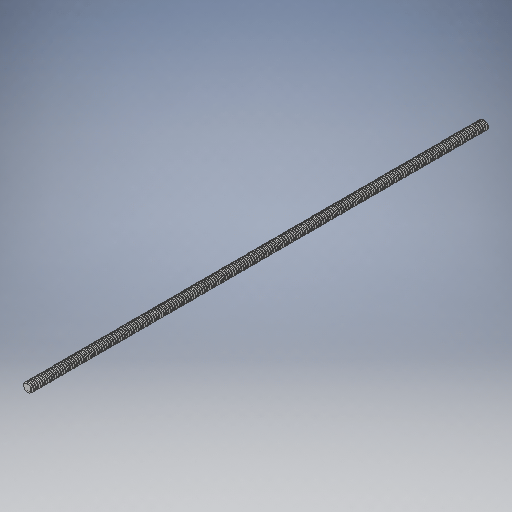
# Autodesk Inventor part: Lead screw 2pitch_8lead_400mm
Saved by Autodesk Inventor 2025.2 (Build 292293000, 293)
## iProperties
Created: 2025-04-06
Part Number: Lead screw 2pitch_8lead_400mm
Material: Generic
Document SubType Name: Modeling
Designer: Tiago
Density: 1 g/cm^3
Appearance: Default
Author: Tiago
Autodesk Inventor part; units mm, degrees
ref_plane "YZ Plane" through (0, 0, 0) normal (1, 0, 0) x (0, 1, 0)
ref_plane "XZ Plane" through (0, 0, 0) normal (0, 1, 0) x (-1, 0, 0)
ref_plane "XY Plane" through (0, 0, 0) normal (0, 0, 1) x (1, 0, 0)
sketch "Sketch1" plane through (0, 0, 0) normal (0, 0, 1) x (1, 0, 0)
  circle A0 centre (0, 0) radius 4
  dimension "Base" = 8
  constraints: 1 centre point, 1 coincident
  measures "Base" diameter of A0
extrude "Extrusion1" add sketch "Sketch1" along normal blind 400
chamfer "Chamfer1" distance 0.3 angle 45 1 edges at (-4, 0, 400)
sketch "Sketch2" plane through (0, 0, 0) normal (0, 1, 0) x (-1, 0, 0)
  line L0 (-4, 399.7) -> (-3.7, 400) projected
  line L1 (-3.7, 400) -> (3.7, 400) projected
  line L2 (3.7, 400) -> (4, 399.7) projected
  line L3 (4, 399.7) -> (4, 0) projected
  line L4 (4, 0) -> (-4, 0) projected
  line L5 (-4, 0) -> (-4, 399.7) projected
  line L6 (4, 400.6339) -> (2.75, 400.6339) construction
  line L7 (2.75, 400.9329) -> (2.75, 400.3349)
  line L8 (4, 401.2679) -> (4, 400)
  line L9 (2.75, 400.3349) -> (4, 400)
  line L10 (2.75, 400.9329) -> (4, 401.2679)
  line L11 (0, 402.735) -> (0, 397.4381) construction
  line L12 (-4, 400.6339) -> (-2.75, 400.6339) construction
  line L13 (-2.75, 400.9329) -> (-2.75, 400.3349)
  line L14 (-4, 401.2679) -> (-4, 400)
  line L15 (-2.75, 400.3349) -> (-4, 400)
  line L16 (-2.75, 400.9329) -> (-4, 401.2679)
  point P0 (0, 0)
  dimension "di" = 1.25
  dimension "d8" = 0.598
  dimension "d12" = 30
  constraints: 22 end point, 6 symmetric about line, 1 collinear, 1 midpoint, 1 parallel, 1 vertical
  measures "di" distance of L6.start L6.end
  measures "d8" distance of L7.start L7.end
  measures "d12" angle of L10 L9
coil "Coil1" sketch "Sketch2" operation cut axis through (0, 0, -10) along (0, 0, -1) pitch 2 turns 202.5 hand right contours L10 L8 L9 L7
sketch "Sketch3" plane through (0, 0, 0) normal (1, 0, 0) x (0, 1, 0)
  line L0 (2.75, 0.4329) -> (2.75, 0) projected
  line L1 (2.75, 0) -> (-4, 0) projected
  line L2 (-2.75, 398.8349) -> (-2.75, 399.4329) projected
  line L3 (-3.7, 400) -> (2.75, 400) projected
  line L4 (2.75, 400) -> (2.75, 399.8349) projected
  line L5 (-2.75, 0.8349) -> (-2.75, 1.4329) projected
  line L6 (-2.75, 2.8349) -> (-2.75, 3.4329) projected
  line L7 (-2.75, 4.8349) -> (-2.75, 5.4329) projected
  line L8 (-2.75, 6.8349) -> (-2.75, 7.4329) projected
  line L9 (-2.75, 8.8349) -> (-2.75, 9.4329) projected
  line L10 (-2.75, 10.8349) -> (-2.75, 11.4329) projected
  line L11 (-2.75, 12.8349) -> (-2.75, 13.4329) projected
  line L12 (-2.75, 14.8349) -> (-2.75, 15.4329) projected
  line L13 (-2.75, 16.8349) -> (-2.75, 17.4329) projected
  line L14 (-2.75, 18.8349) -> (-2.75, 19.4329) projected
  line L15 (-2.75, 20.8349) -> (-2.75, 21.4329) projected
  line L16 (-2.75, 22.8349) -> (-2.75, 23.4329) projected
  line L17 (-2.75, 24.8349) -> (-2.75, 25.4329) projected
  line L18 (-2.75, 26.8349) -> (-2.75, 27.4329) projected
  line L19 (-2.75, 28.8349) -> (-2.75, 29.4329) projected
  line L20 (-2.75, 30.8349) -> (-2.75, 31.4329) projected
  line L21 (-2.75, 32.8349) -> (-2.75, 33.4329) projected
  line L22 (-2.75, 34.8349) -> (-2.75, 35.4329) projected
  line L23 (-2.75, 36.8349) -> (-2.75, 37.4329) projected
  line L24 (-2.75, 38.8349) -> (-2.75, 39.4329) projected
  line L25 (-2.75, 40.8349) -> (-2.75, 41.4329) projected
  line L26 (-2.75, 42.8349) -> (-2.75, 43.4329) projected
  line L27 (-2.75, 44.8349) -> (-2.75, 45.4329) projected
  line L28 (-2.75, 46.8349) -> (-2.75, 47.4329) projected
  line L29 (-2.75, 48.8349) -> (-2.75, 49.4329) projected
  line L30 (-2.75, 50.8349) -> (-2.75, 51.4329) projected
  line L31 (-2.75, 52.8349) -> (-2.75, 53.4329) projected
  line L32 (-2.75, 54.8349) -> (-2.75, 55.4329) projected
  line L33 (-2.75, 56.8349) -> (-2.75, 57.4329) projected
  line L34 (-2.75, 58.8349) -> (-2.75, 59.4329) projected
  line L35 (-2.75, 60.8349) -> (-2.75, 61.4329) projected
  line L36 (-2.75, 62.8349) -> (-2.75, 63.4329) projected
  line L37 (-2.75, 64.8349) -> (-2.75, 65.4329) projected
  line L38 (-2.75, 66.8349) -> (-2.75, 67.4329) projected
  line L39 (-2.75, 68.8349) -> (-2.75, 69.4329) projected
  line L40 (-2.75, 70.8349) -> (-2.75, 71.4329) projected
  line L41 (-2.75, 72.8349) -> (-2.75, 73.4329) projected
  line L42 (-2.75, 74.8349) -> (-2.75, 75.4329) projected
  line L43 (-2.75, 76.8349) -> (-2.75, 77.4329) projected
  line L44 (-2.75, 78.8349) -> (-2.75, 79.4329) projected
  line L45 (-2.75, 80.8349) -> (-2.75, 81.4329) projected
  line L46 (-2.75, 82.8349) -> (-2.75, 83.4329) projected
  line L47 (-2.75, 84.8349) -> (-2.75, 85.4329) projected
  line L48 (-2.75, 86.8349) -> (-2.75, 87.4329) projected
  line L49 (-2.75, 88.8349) -> (-2.75, 89.4329) projected
  line L50 (-2.75, 90.8349) -> (-2.75, 91.4329) projected
  line L51 (-2.75, 92.8349) -> (-2.75, 93.4329) projected
  line L52 (-2.75, 94.8349) -> (-2.75, 95.4329) projected
  line L53 (-2.75, 96.8349) -> (-2.75, 97.4329) projected
  line L54 (-2.75, 98.8349) -> (-2.75, 99.4329) projected
  line L55 (-2.75, 100.8349) -> (-2.75, 101.4329) projected
  line L56 (-2.75, 102.8349) -> (-2.75, 103.4329) projected
  line L57 (-2.75, 104.8349) -> (-2.75, 105.4329) projected
  line L58 (-2.75, 106.8349) -> (-2.75, 107.4329) projected
  line L59 (-2.75, 108.8349) -> (-2.75, 109.4329) projected
  line L60 (-2.75, 110.8349) -> (-2.75, 111.4329) projected
  line L61 (-2.75, 112.8349) -> (-2.75, 113.4329) projected
  line L62 (-2.75, 114.8349) -> (-2.75, 115.4329) projected
  line L63 (-2.75, 116.8349) -> (-2.75, 117.4329) projected
  line L64 (-2.75, 118.8349) -> (-2.75, 119.4329) projected
  line L65 (-2.75, 120.8349) -> (-2.75, 121.4329) projected
  line L66 (-2.75, 122.8349) -> (-2.75, 123.4329) projected
  line L67 (-2.75, 124.8349) -> (-2.75, 125.4329) projected
  line L68 (-2.75, 126.8349) -> (-2.75, 127.4329) projected
  line L69 (-2.75, 128.8349) -> (-2.75, 129.4329) projected
  line L70 (-2.75, 130.8349) -> (-2.75, 131.4329) projected
  line L71 (-2.75, 132.8349) -> (-2.75, 133.4329) projected
  line L72 (-2.75, 134.8349) -> (-2.75, 135.4329) projected
  line L73 (-2.75, 136.8349) -> (-2.75, 137.4329) projected
  line L74 (-2.75, 138.8349) -> (-2.75, 139.4329) projected
  line L75 (-2.75, 140.8349) -> (-2.75, 141.4329) projected
  line L76 (-2.75, 142.8349) -> (-2.75, 143.4329) projected
  line L77 (-2.75, 144.8349) -> (-2.75, 145.4329) projected
  line L78 (-2.75, 146.8349) -> (-2.75, 147.4329) projected
  line L79 (-2.75, 148.8349) -> (-2.75, 149.4329) projected
  line L80 (-2.75, 150.8349) -> (-2.75, 151.4329) projected
  line L81 (-2.75, 152.8349) -> (-2.75, 153.4329) projected
  line L82 (-2.75, 154.8349) -> (-2.75, 155.4329) projected
  line L83 (-2.75, 156.8349) -> (-2.75, 157.4329) projected
  line L84 (-2.75, 158.8349) -> (-2.75, 159.4329) projected
  line L85 (-2.75, 160.8349) -> (-2.75, 161.4329) projected
  line L86 (-2.75, 162.8349) -> (-2.75, 163.4329) projected
  line L87 (-2.75, 164.8349) -> (-2.75, 165.4329) projected
  line L88 (-2.75, 166.8349) -> (-2.75, 167.4329) projected
  line L89 (-2.75, 168.8349) -> (-2.75, 169.4329) projected
  line L90 (-2.75, 170.8349) -> (-2.75, 171.4329) projected
  line L91 (-2.75, 172.8349) -> (-2.75, 173.4329) projected
  line L92 (-2.75, 174.8349) -> (-2.75, 175.4329) projected
  line L93 (-2.75, 176.8349) -> (-2.75, 177.4329) projected
  line L94 (-2.75, 178.8349) -> (-2.75, 179.4329) projected
  line L95 (-2.75, 180.8349) -> (-2.75, 181.4329) projected
  line L96 (-2.75, 182.8349) -> (-2.75, 183.4329) projected
  line L97 (-2.75, 184.8349) -> (-2.75, 185.4329) projected
  line L98 (-2.75, 186.8349) -> (-2.75, 187.4329) projected
  line L99 (-2.75, 188.8349) -> (-2.75, 189.4329) projected
  line L100 (-2.75, 190.8349) -> (-2.75, 191.4329) projected
  line L101 (-2.75, 192.8349) -> (-2.75, 193.4329) projected
  line L102 (-2.75, 194.8349) -> (-2.75, 195.4329) projected
  line L103 (-2.75, 196.8349) -> (-2.75, 197.4329) projected
  line L104 (-2.75, 198.8349) -> (-2.75, 199.4329) projected
  line L105 (-2.75, 200.8349) -> (-2.75, 201.4329) projected
  line L106 (-2.75, 202.8349) -> (-2.75, 203.4329) projected
  line L107 (-2.75, 204.8349) -> (-2.75, 205.4329) projected
  line L108 (-2.75, 206.8349) -> (-2.75, 207.4329) projected
  line L109 (-2.75, 208.8349) -> (-2.75, 209.4329) projected
  line L110 (-2.75, 210.8349) -> (-2.75, 211.4329) projected
  line L111 (-2.75, 212.8349) -> (-2.75, 213.4329) projected
  line L112 (-2.75, 214.8349) -> (-2.75, 215.4329) projected
  line L113 (-2.75, 216.8349) -> (-2.75, 217.4329) projected
  line L114 (-2.75, 218.8349) -> (-2.75, 219.4329) projected
  line L115 (-2.75, 220.8349) -> (-2.75, 221.4329) projected
  line L116 (-2.75, 222.8349) -> (-2.75, 223.4329) projected
  line L117 (-2.75, 224.8349) -> (-2.75, 225.4329) projected
  line L118 (-2.75, 226.8349) -> (-2.75, 227.4329) projected
  line L119 (-2.75, 228.8349) -> (-2.75, 229.4329) projected
  line L120 (-2.75, 230.8349) -> (-2.75, 231.4329) projected
  line L121 (-2.75, 232.8349) -> (-2.75, 233.4329) projected
  line L122 (-2.75, 234.8349) -> (-2.75, 235.4329) projected
  line L123 (-2.75, 236.8349) -> (-2.75, 237.4329) projected
  line L124 (-2.75, 238.8349) -> (-2.75, 239.4329) projected
  line L125 (-2.75, 240.8349) -> (-2.75, 241.4329) projected
  line L126 (-2.75, 242.8349) -> (-2.75, 243.4329) projected
  line L127 (-2.75, 244.8349) -> (-2.75, 245.4329) projected
  line L128 (-2.75, 246.8349) -> (-2.75, 247.4329) projected
  line L129 (-2.75, 248.8349) -> (-2.75, 249.4329) projected
  line L130 (-2.75, 250.8349) -> (-2.75, 251.4329) projected
  line L131 (-2.75, 252.8349) -> (-2.75, 253.4329) projected
  line L132 (-2.75, 254.8349) -> (-2.75, 255.4329) projected
  line L133 (-2.75, 256.8349) -> (-2.75, 257.4329) projected
  line L134 (-2.75, 258.8349) -> (-2.75, 259.4329) projected
  line L135 (-2.75, 260.8349) -> (-2.75, 261.4329) projected
  line L136 (-2.75, 262.8349) -> (-2.75, 263.4329) projected
  line L137 (-2.75, 264.8349) -> (-2.75, 265.4329) projected
  line L138 (-2.75, 266.8349) -> (-2.75, 267.4329) projected
  line L139 (-2.75, 268.8349) -> (-2.75, 269.4329) projected
  line L140 (-2.75, 270.8349) -> (-2.75, 271.4329) projected
  line L141 (-2.75, 272.8349) -> (-2.75, 273.4329) projected
  line L142 (-2.75, 274.8349) -> (-2.75, 275.4329) projected
  line L143 (-2.75, 276.8349) -> (-2.75, 277.4329) projected
  line L144 (-2.75, 278.8349) -> (-2.75, 279.4329) projected
  line L145 (-2.75, 280.8349) -> (-2.75, 281.4329) projected
  line L146 (-2.75, 282.8349) -> (-2.75, 283.4329) projected
  line L147 (-2.75, 284.8349) -> (-2.75, 285.4329) projected
  line L148 (-2.75, 286.8349) -> (-2.75, 287.4329) projected
  line L149 (-2.75, 288.8349) -> (-2.75, 289.4329) projected
  line L150 (-2.75, 290.8349) -> (-2.75, 291.4329) projected
  line L151 (-2.75, 292.8349) -> (-2.75, 293.4329) projected
  line L152 (-2.75, 294.8349) -> (-2.75, 295.4329) projected
  line L153 (-2.75, 296.8349) -> (-2.75, 297.4329) projected
  line L154 (-2.75, 298.8349) -> (-2.75, 299.4329) projected
  line L155 (-2.75, 300.8349) -> (-2.75, 301.4329) projected
  line L156 (-2.75, 302.8349) -> (-2.75, 303.4329) projected
  line L157 (-2.75, 304.8349) -> (-2.75, 305.4329) projected
  line L158 (-2.75, 306.8349) -> (-2.75, 307.4329) projected
  line L159 (-2.75, 308.8349) -> (-2.75, 309.4329) projected
  line L160 (-2.75, 310.8349) -> (-2.75, 311.4329) projected
  line L161 (-2.75, 312.8349) -> (-2.75, 313.4329) projected
  line L162 (-2.75, 314.8349) -> (-2.75, 315.4329) projected
  line L163 (-2.75, 316.8349) -> (-2.75, 317.4329) projected
  line L164 (-2.75, 318.8349) -> (-2.75, 319.4329) projected
  line L165 (-2.75, 320.8349) -> (-2.75, 321.4329) projected
  line L166 (-2.75, 322.8349) -> (-2.75, 323.4329) projected
  line L167 (-2.75, 324.8349) -> (-2.75, 325.4329) projected
  line L168 (-2.75, 326.8349) -> (-2.75, 327.4329) projected
  line L169 (-2.75, 328.8349) -> (-2.75, 329.4329) projected
  line L170 (-2.75, 330.8349) -> (-2.75, 331.4329) projected
  line L171 (-2.75, 332.8349) -> (-2.75, 333.4329) projected
  line L172 (-2.75, 334.8349) -> (-2.75, 335.4329) projected
  line L173 (-2.75, 336.8349) -> (-2.75, 337.4329) projected
  line L174 (-2.75, 338.8349) -> (-2.75, 339.4329) projected
  line L175 (-2.75, 340.8349) -> (-2.75, 341.4329) projected
  line L176 (-2.75, 342.8349) -> (-2.75, 343.4329) projected
  line L177 (-2.75, 344.8349) -> (-2.75, 345.4329) projected
  line L178 (-2.75, 346.8349) -> (-2.75, 347.4329) projected
  line L179 (-2.75, 348.8349) -> (-2.75, 349.4329) projected
  line L180 (-2.75, 350.8349) -> (-2.75, 351.4329) projected
  line L181 (-2.75, 352.8349) -> (-2.75, 353.4329) projected
  line L182 (-2.75, 354.8349) -> (-2.75, 355.4329) projected
  line L183 (-2.75, 356.8349) -> (-2.75, 357.4329) projected
  line L184 (-2.75, 358.8349) -> (-2.75, 359.4329) projected
  line L185 (-2.75, 360.8349) -> (-2.75, 361.4329) projected
  line L186 (-2.75, 362.8349) -> (-2.75, 363.4329) projected
  line L187 (-2.75, 364.8349) -> (-2.75, 365.4329) projected
  line L188 (-2.75, 366.8349) -> (-2.75, 367.4329) projected
  line L189 (-2.75, 368.8349) -> (-2.75, 369.4329) projected
  line L190 (-2.75, 370.8349) -> (-2.75, 371.4329) projected
  line L191 (-2.75, 372.8349) -> (-2.75, 373.4329) projected
  line L192 (-2.75, 374.8349) -> (-2.75, 375.4329) projected
  line L193 (-2.75, 376.8349) -> (-2.75, 377.4329) projected
  line L194 (-2.75, 378.8349) -> (-2.75, 379.4329) projected
  line L195 (-2.75, 380.8349) -> (-2.75, 381.4329) projected
  line L196 (-2.75, 382.8349) -> (-2.75, 383.4329) projected
  line L197 (-2.75, 384.8349) -> (-2.75, 385.4329) projected
  line L198 (-2.75, 386.8349) -> (-2.75, 387.4329) projected
  line L199 (-2.75, 388.8349) -> (-2.75, 389.4329) projected
  line L200 (-2.75, 390.8349) -> (-2.75, 391.4329) projected
  line L201 (-2.75, 392.8349) -> (-2.75, 393.4329) projected
  line L202 (-2.75, 394.8349) -> (-2.75, 395.4329) projected
  line L203 (-2.75, 396.8349) -> (-2.75, 397.4329) projected
  line L204 (2.7534, 400.6412) -> (4.0034, 400.6412) construction
  line L205 (4.0034, 400.9402) -> (4.0034, 400.3422)
  line L206 (2.7534, 401.2752) -> (2.7534, 400.0073)
  line L207 (4.0034, 400.3422) -> (2.7534, 400.0073)
  line L208 (4.0034, 400.9402) -> (2.7534, 401.2752)
  line L209 (0, 399.0551) -> (0, 402.6988)
  line L210 (-3.9465, 399.7535) -> (-3.7, 400) projected
  line L211 (4, 399.5) -> (4, 398.7679) projected
  line L212 (2.75, 398.4329) -> (2.75, 397.8349) projected
  line L213 (4, 397.5) -> (4, 396.7679) projected
  line L214 (2.75, 396.4329) -> (2.75, 395.8349) projected
  line L215 (4, 395.5) -> (4, 394.7679) projected
  line L216 (2.75, 394.4329) -> (2.75, 393.8349) projected
  line L217 (4, 393.5) -> (4, 392.7679) projected
  line L218 (2.75, 392.4329) -> (2.75, 391.8349) projected
  line L219 (4, 391.5) -> (4, 390.7679) projected
  line L220 (2.75, 390.4329) -> (2.75, 389.8349) projected
  line L221 (4, 389.5) -> (4, 388.7679) projected
  line L222 (2.75, 388.4329) -> (2.75, 387.8349) projected
  line L223 (4, 387.5) -> (4, 386.7679) projected
  line L224 (2.75, 386.4329) -> (2.75, 385.8349) projected
  line L225 (4, 385.5) -> (4, 384.7679) projected
  line L226 (2.75, 384.4329) -> (2.75, 383.8349) projected
  line L227 (4, 383.5) -> (4, 382.7679) projected
  line L228 (2.75, 382.4329) -> (2.75, 381.8349) projected
  line L229 (4, 381.5) -> (4, 380.7679) projected
  line L230 (2.75, 380.4329) -> (2.75, 379.8349) projected
  line L231 (4, 379.5) -> (4, 378.7679) projected
  line L232 (2.75, 378.4329) -> (2.75, 377.8349) projected
  line L233 (4, 377.5) -> (4, 376.7679) projected
  line L234 (2.75, 376.4329) -> (2.75, 375.8349) projected
  line L235 (4, 375.5) -> (4, 374.7679) projected
  line L236 (2.75, 374.4329) -> (2.75, 373.8349) projected
  line L237 (4, 373.5) -> (4, 372.7679) projected
  line L238 (2.75, 372.4329) -> (2.75, 371.8349) projected
  line L239 (4, 371.5) -> (4, 370.7679) projected
  line L240 (2.75, 370.4329) -> (2.75, 369.8349) projected
  line L241 (4, 369.5) -> (4, 368.7679) projected
  line L242 (2.75, 368.4329) -> (2.75, 367.8349) projected
  line L243 (4, 367.5) -> (4, 366.7679) projected
  line L244 (2.75, 366.4329) -> (2.75, 365.8349) projected
  line L245 (4, 365.5) -> (4, 364.7679) projected
  line L246 (2.75, 364.4329) -> (2.75, 363.8349) projected
  line L247 (4, 363.5) -> (4, 362.7679) projected
  line L248 (2.75, 362.4329) -> (2.75, 361.8349) projected
  line L249 (4, 361.5) -> (4, 360.7679) projected
  line L250 (2.75, 360.4329) -> (2.75, 359.8349) projected
  line L251 (4, 359.5) -> (4, 358.7679) projected
  line L252 (2.75, 358.4329) -> (2.75, 357.8349) projected
  line L253 (4, 357.5) -> (4, 356.7679) projected
  line L254 (2.75, 356.4329) -> (2.75, 355.8349) projected
  line L255 (4, 355.5) -> (4, 354.7679) projected
  line L256 (2.75, 354.4329) -> (2.75, 353.8349) projected
  line L257 (4, 353.5) -> (4, 352.7679) projected
  line L258 (2.75, 352.4329) -> (2.75, 351.8349) projected
  line L259 (4, 351.5) -> (4, 350.7679) projected
  line L260 (2.75, 350.4329) -> (2.75, 349.8349) projected
  line L261 (4, 349.5) -> (4, 348.7679) projected
  line L262 (2.75, 348.4329) -> (2.75, 347.8349) projected
  line L263 (4, 347.5) -> (4, 346.7679) projected
  line L264 (2.75, 346.4329) -> (2.75, 345.8349) projected
  line L265 (4, 345.5) -> (4, 344.7679) projected
  line L266 (2.75, 344.4329) -> (2.75, 343.8349) projected
  line L267 (4, 343.5) -> (4, 342.7679) projected
  line L268 (2.75, 342.4329) -> (2.75, 341.8349) projected
  line L269 (4, 341.5) -> (4, 340.7679) projected
  line L270 (2.75, 340.4329) -> (2.75, 339.8349) projected
  line L271 (4, 339.5) -> (4, 338.7679) projected
  line L272 (2.75, 338.4329) -> (2.75, 337.8349) projected
  line L273 (4, 337.5) -> (4, 336.7679) projected
  line L274 (2.75, 336.4329) -> (2.75, 335.8349) projected
  line L275 (4, 335.5) -> (4, 334.7679) projected
  line L276 (2.75, 334.4329) -> (2.75, 333.8349) projected
  line L277 (4, 333.5) -> (4, 332.7679) projected
  line L278 (2.75, 332.4329) -> (2.75, 331.8349) projected
  line L279 (4, 331.5) -> (4, 330.7679) projected
  line L280 (2.75, 330.4329) -> (2.75, 329.8349) projected
  line L281 (4, 329.5) -> (4, 328.7679) projected
  line L282 (2.75, 328.4329) -> (2.75, 327.8349) projected
  line L283 (4, 327.5) -> (4, 326.7679) projected
  line L284 (2.75, 326.4329) -> (2.75, 325.8349) projected
  line L285 (4, 325.5) -> (4, 324.7679) projected
  line L286 (2.75, 324.4329) -> (2.75, 323.8349) projected
  line L287 (4, 323.5) -> (4, 322.7679) projected
  line L288 (2.75, 322.4329) -> (2.75, 321.8349) projected
  line L289 (4, 321.5) -> (4, 320.7679) projected
  line L290 (2.75, 320.4329) -> (2.75, 319.8349) projected
  line L291 (4, 319.5) -> (4, 318.7679) projected
  line L292 (2.75, 318.4329) -> (2.75, 317.8349) projected
  line L293 (4, 317.5) -> (4, 316.7679) projected
  line L294 (2.75, 316.4329) -> (2.75, 315.8349) projected
  line L295 (4, 315.5) -> (4, 314.7679) projected
  line L296 (2.75, 314.4329) -> (2.75, 313.8349) projected
  line L297 (4, 313.5) -> (4, 312.7679) projected
  line L298 (2.75, 312.4329) -> (2.75, 311.8349) projected
  line L299 (4, 311.5) -> (4, 310.7679) projected
  line L300 (2.75, 310.4329) -> (2.75, 309.8349) projected
  line L301 (4, 309.5) -> (4, 308.7679) projected
  line L302 (2.75, 308.4329) -> (2.75, 307.8349) projected
  line L303 (4, 307.5) -> (4, 306.7679) projected
  line L304 (2.75, 306.4329) -> (2.75, 305.8349) projected
  line L305 (4, 305.5) -> (4, 304.7679) projected
  line L306 (2.75, 304.4329) -> (2.75, 303.8349) projected
  line L307 (4, 303.5) -> (4, 302.7679) projected
  line L308 (2.75, 302.4329) -> (2.75, 301.8349) projected
  line L309 (4, 301.5) -> (4, 300.7679) projected
  line L310 (2.75, 300.4329) -> (2.75, 299.8349) projected
  line L311 (4, 299.5) -> (4, 298.7679) projected
  line L312 (2.75, 298.4329) -> (2.75, 297.8349) projected
  line L313 (4, 297.5) -> (4, 296.7679) projected
  line L314 (2.75, 296.4329) -> (2.75, 295.8349) projected
  line L315 (4, 295.5) -> (4, 294.7679) projected
  line L316 (2.75, 294.4329) -> (2.75, 293.8349) projected
  line L317 (4, 293.5) -> (4, 292.7679) projected
  line L318 (2.75, 292.4329) -> (2.75, 291.8349) projected
  line L319 (4, 291.5) -> (4, 290.7679) projected
  line L320 (2.75, 290.4329) -> (2.75, 289.8349) projected
  line L321 (4, 289.5) -> (4, 288.7679) projected
  line L322 (2.75, 288.4329) -> (2.75, 287.8349) projected
  line L323 (4, 287.5) -> (4, 286.7679) projected
  line L324 (2.75, 286.4329) -> (2.75, 285.8349) projected
  line L325 (4, 285.5) -> (4, 284.7679) projected
  line L326 (2.75, 284.4329) -> (2.75, 283.8349) projected
  line L327 (4, 283.5) -> (4, 282.7679) projected
  line L328 (2.75, 282.4329) -> (2.75, 281.8349) projected
  line L329 (4, 281.5) -> (4, 280.7679) projected
  line L330 (2.75, 280.4329) -> (2.75, 279.8349) projected
  line L331 (4, 279.5) -> (4, 278.7679) projected
  line L332 (2.75, 278.4329) -> (2.75, 277.8349) projected
  line L333 (4, 277.5) -> (4, 276.7679) projected
  line L334 (2.75, 276.4329) -> (2.75, 275.8349) projected
  line L335 (4, 275.5) -> (4, 274.7679) projected
  line L336 (2.75, 274.4329) -> (2.75, 273.8349) projected
  line L337 (4, 273.5) -> (4, 272.7679) projected
  line L338 (2.75, 272.4329) -> (2.75, 271.8349) projected
  line L339 (4, 271.5) -> (4, 270.7679) projected
  line L340 (2.75, 270.4329) -> (2.75, 269.8349) projected
  line L341 (4, 269.5) -> (4, 268.7679) projected
  line L342 (2.75, 268.4329) -> (2.75, 267.8349) projected
  line L343 (4, 267.5) -> (4, 266.7679) projected
  line L344 (2.75, 266.4329) -> (2.75, 265.8349) projected
  line L345 (4, 265.5) -> (4, 264.7679) projected
  line L346 (2.75, 264.4329) -> (2.75, 263.8349) projected
  line L347 (4, 263.5) -> (4, 262.7679) projected
  line L348 (2.75, 262.4329) -> (2.75, 261.8349) projected
  line L349 (4, 261.5) -> (4, 260.7679) projected
  line L350 (2.75, 260.4329) -> (2.75, 259.8349) projected
  line L351 (4, 259.5) -> (4, 258.7679) projected
  line L352 (2.75, 258.4329) -> (2.75, 257.8349) projected
  line L353 (4, 257.5) -> (4, 256.7679) projected
  line L354 (2.75, 256.4329) -> (2.75, 255.8349) projected
  line L355 (4, 255.5) -> (4, 254.7679) projected
  line L356 (2.75, 254.4329) -> (2.75, 253.8349) projected
  line L357 (4, 253.5) -> (4, 252.7679) projected
  line L358 (2.75, 252.4329) -> (2.75, 251.8349) projected
  line L359 (4, 251.5) -> (4, 250.7679) projected
  line L360 (2.75, 250.4329) -> (2.75, 249.8349) projected
  line L361 (4, 249.5) -> (4, 248.7679) projected
  line L362 (2.75, 248.4329) -> (2.75, 247.8349) projected
  line L363 (4, 247.5) -> (4, 246.7679) projected
  line L364 (2.75, 246.4329) -> (2.75, 245.8349) projected
  line L365 (4, 245.5) -> (4, 244.7679) projected
  line L366 (2.75, 244.4329) -> (2.75, 243.8349) projected
  line L367 (4, 243.5) -> (4, 242.7679) projected
  line L368 (2.75, 242.4329) -> (2.75, 241.8349) projected
  line L369 (4, 241.5) -> (4, 240.7679) projected
  line L370 (2.75, 240.4329) -> (2.75, 239.8349) projected
  line L371 (4, 239.5) -> (4, 238.7679) projected
  line L372 (2.75, 238.4329) -> (2.75, 237.8349) projected
  line L373 (4, 237.5) -> (4, 236.7679) projected
  line L374 (2.75, 236.4329) -> (2.75, 235.8349) projected
  line L375 (4, 235.5) -> (4, 234.7679) projected
  line L376 (2.75, 234.4329) -> (2.75, 233.8349) projected
  line L377 (4, 233.5) -> (4, 232.7679) projected
  line L378 (2.75, 232.4329) -> (2.75, 231.8349) projected
  line L379 (4, 231.5) -> (4, 230.7679) projected
  line L380 (2.75, 230.4329) -> (2.75, 229.8349) projected
  line L381 (4, 229.5) -> (4, 228.7679) projected
  line L382 (2.75, 228.4329) -> (2.75, 227.8349) projected
  line L383 (4, 227.5) -> (4, 226.7679) projected
  line L384 (2.75, 226.4329) -> (2.75, 225.8349) projected
  line L385 (4, 225.5) -> (4, 224.7679) projected
  line L386 (2.75, 224.4329) -> (2.75, 223.8349) projected
  line L387 (4, 223.5) -> (4, 222.7679) projected
  line L388 (2.75, 222.4329) -> (2.75, 221.8349) projected
  line L389 (4, 221.5) -> (4, 220.7679) projected
  line L390 (2.75, 220.4329) -> (2.75, 219.8349) projected
  line L391 (4, 219.5) -> (4, 218.7679) projected
  line L392 (2.75, 218.4329) -> (2.75, 217.8349) projected
  line L393 (4, 217.5) -> (4, 216.7679) projected
  line L394 (2.75, 216.4329) -> (2.75, 215.8349) projected
  line L395 (4, 215.5) -> (4, 214.7679) projected
  line L396 (2.75, 214.4329) -> (2.75, 213.8349) projected
  line L397 (4, 213.5) -> (4, 212.7679) projected
  line L398 (2.75, 212.4329) -> (2.75, 211.8349) projected
  line L399 (4, 211.5) -> (4, 210.7679) projected
  line L400 (2.75, 210.4329) -> (2.75, 209.8349) projected
  line L401 (4, 209.5) -> (4, 208.7679) projected
  line L402 (2.75, 208.4329) -> (2.75, 207.8349) projected
  line L403 (4, 207.5) -> (4, 206.7679) projected
  line L404 (2.75, 206.4329) -> (2.75, 205.8349) projected
  line L405 (4, 205.5) -> (4, 204.7679) projected
  line L406 (2.75, 204.4329) -> (2.75, 203.8349) projected
  line L407 (4, 203.5) -> (4, 202.7679) projected
  line L408 (2.75, 202.4329) -> (2.75, 201.8349) projected
  line L409 (4, 201.5) -> (4, 200.7679) projected
  line L410 (2.75, 200.4329) -> (2.75, 199.8349) projected
  line L411 (4, 199.5) -> (4, 198.7679) projected
  line L412 (2.75, 198.4329) -> (2.75, 197.8349) projected
  line L413 (4, 197.5) -> (4, 196.7679) projected
  line L414 (2.75, 196.4329) -> (2.75, 195.8349) projected
  line L415 (4, 195.5) -> (4, 194.7679) projected
  line L416 (2.75, 194.4329) -> (2.75, 193.8349) projected
  line L417 (4, 193.5) -> (4, 192.7679) projected
  line L418 (2.75, 192.4329) -> (2.75, 191.8349) projected
  line L419 (4, 191.5) -> (4, 190.7679) projected
  line L420 (2.75, 190.4329) -> (2.75, 189.8349) projected
  line L421 (4, 189.5) -> (4, 188.7679) projected
  line L422 (2.75, 188.4329) -> (2.75, 187.8349) projected
  line L423 (4, 187.5) -> (4, 186.7679) projected
  line L424 (2.75, 186.4329) -> (2.75, 185.8349) projected
  line L425 (4, 185.5) -> (4, 184.7679) projected
  line L426 (2.75, 184.4329) -> (2.75, 183.8349) projected
  line L427 (4, 183.5) -> (4, 182.7679) projected
  line L428 (2.75, 182.4329) -> (2.75, 181.8349) projected
  line L429 (4, 181.5) -> (4, 180.7679) projected
  line L430 (2.75, 180.4329) -> (2.75, 179.8349) projected
  line L431 (4, 179.5) -> (4, 178.7679) projected
  line L432 (2.75, 178.4329) -> (2.75, 177.8349) projected
  line L433 (4, 177.5) -> (4, 176.7679) projected
  line L434 (2.75, 176.4329) -> (2.75, 175.8349) projected
  line L435 (4, 175.5) -> (4, 174.7679) projected
  line L436 (2.75, 174.4329) -> (2.75, 173.8349) projected
  line L437 (4, 173.5) -> (4, 172.7679) projected
  line L438 (2.75, 172.4329) -> (2.75, 171.8349) projected
  line L439 (4, 171.5) -> (4, 170.7679) projected
  line L440 (2.75, 170.4329) -> (2.75, 169.8349) projected
  line L441 (4, 169.5) -> (4, 168.7679) projected
  line L442 (2.75, 168.4329) -> (2.75, 167.8349) projected
  line L443 (4, 167.5) -> (4, 166.7679) projected
  line L444 (2.75, 166.4329) -> (2.75, 165.8349) projected
  line L445 (4, 165.5) -> (4, 164.7679) projected
  line L446 (2.75, 164.4329) -> (2.75, 163.8349) projected
  line L447 (4, 163.5) -> (4, 162.7679) projected
  line L448 (2.75, 162.4329) -> (2.75, 161.8349) projected
  line L449 (4, 161.5) -> (4, 160.7679) projected
  line L450 (2.75, 160.4329) -> (2.75, 159.8349) projected
  line L451 (4, 159.5) -> (4, 158.7679) projected
  line L452 (2.75, 158.4329) -> (2.75, 157.8349) projected
  line L453 (4, 157.5) -> (4, 156.7679) projected
  line L454 (2.75, 156.4329) -> (2.75, 155.8349) projected
  line L455 (4, 155.5) -> (4, 154.7679) projected
  line L456 (2.75, 154.4329) -> (2.75, 153.8349) projected
  line L457 (4, 153.5) -> (4, 152.7679) projected
  line L458 (2.75, 152.4329) -> (2.75, 151.8349) projected
  line L459 (4, 151.5) -> (4, 150.7679) projected
  line L460 (2.75, 150.4329) -> (2.75, 149.8349) projected
  line L461 (4, 149.5) -> (4, 148.7679) projected
  line L462 (2.75, 148.4329) -> (2.75, 147.8349) projected
  line L463 (4, 147.5) -> (4, 146.7679) projected
  line L464 (2.75, 146.4329) -> (2.75, 145.8349) projected
  line L465 (4, 145.5) -> (4, 144.7679) projected
  line L466 (2.75, 144.4329) -> (2.75, 143.8349) projected
  line L467 (4, 143.5) -> (4, 142.7679) projected
  line L468 (2.75, 142.4329) -> (2.75, 141.8349) projected
  line L469 (4, 141.5) -> (4, 140.7679) projected
  line L470 (2.75, 140.4329) -> (2.75, 139.8349) projected
  line L471 (4, 139.5) -> (4, 138.7679) projected
  line L472 (2.75, 138.4329) -> (2.75, 137.8349) projected
  line L473 (4, 137.5) -> (4, 136.7679) projected
  line L474 (2.75, 136.4329) -> (2.75, 135.8349) projected
  line L475 (4, 135.5) -> (4, 134.7679) projected
  line L476 (2.75, 134.4329) -> (2.75, 133.8349) projected
  line L477 (4, 133.5) -> (4, 132.7679) projected
  line L478 (2.75, 132.4329) -> (2.75, 131.8349) projected
  line L479 (4, 131.5) -> (4, 130.7679) projected
  line L480 (2.75, 130.4329) -> (2.75, 129.8349) projected
  line L481 (4, 129.5) -> (4, 128.7679) projected
  line L482 (2.75, 128.4329) -> (2.75, 127.8349) projected
  line L483 (4, 127.5) -> (4, 126.7679) projected
  line L484 (2.75, 126.4329) -> (2.75, 125.8349) projected
  line L485 (4, 125.5) -> (4, 124.7679) projected
  line L486 (2.75, 124.4329) -> (2.75, 123.8349) projected
  line L487 (4, 123.5) -> (4, 122.7679) projected
  line L488 (2.75, 122.4329) -> (2.75, 121.8349) projected
  line L489 (4, 121.5) -> (4, 120.7679) projected
  line L490 (2.75, 120.4329) -> (2.75, 119.8349) projected
  line L491 (4, 119.5) -> (4, 118.7679) projected
  line L492 (2.75, 118.4329) -> (2.75, 117.8349) projected
  line L493 (4, 117.5) -> (4, 116.7679) projected
  line L494 (2.75, 116.4329) -> (2.75, 115.8349) projected
  line L495 (4, 115.5) -> (4, 114.7679) projected
  line L496 (2.75, 114.4329) -> (2.75, 113.8349) projected
  line L497 (4, 113.5) -> (4, 112.7679) projected
  line L498 (2.75, 112.4329) -> (2.75, 111.8349) projected
  line L499 (4, 111.5) -> (4, 110.7679) projected
  line L500 (2.75, 110.4329) -> (2.75, 109.8349) projected
  line L501 (4, 109.5) -> (4, 108.7679) projected
  line L502 (2.75, 108.4329) -> (2.75, 107.8349) projected
  line L503 (4, 107.5) -> (4, 106.7679) projected
  line L504 (2.75, 106.4329) -> (2.75, 105.8349) projected
  line L505 (4, 105.5) -> (4, 104.7679) projected
  line L506 (2.75, 104.4329) -> (2.75, 103.8349) projected
  line L507 (4, 103.5) -> (4, 102.7679) projected
  line L508 (2.75, 102.4329) -> (2.75, 101.8349) projected
  line L509 (4, 101.5) -> (4, 100.7679) projected
  line L510 (2.75, 100.4329) -> (2.75, 99.8349) projected
  line L511 (4, 99.5) -> (4, 98.7679) projected
  line L512 (2.75, 98.4329) -> (2.75, 97.8349) projected
  line L513 (4, 97.5) -> (4, 96.7679) projected
  line L514 (2.75, 96.4329) -> (2.75, 95.8349) projected
  line L515 (4, 95.5) -> (4, 94.7679) projected
  line L516 (2.75, 94.4329) -> (2.75, 93.8349) projected
  line L517 (4, 93.5) -> (4, 92.7679) projected
  line L518 (2.75, 92.4329) -> (2.75, 91.8349) projected
  line L519 (4, 91.5) -> (4, 90.7679) projected
  line L520 (2.75, 90.4329) -> (2.75, 89.8349) projected
  line L521 (4, 89.5) -> (4, 88.7679) projected
  line L522 (2.75, 88.4329) -> (2.75, 87.8349) projected
  line L523 (4, 87.5) -> (4, 86.7679) projected
  line L524 (2.75, 86.4329) -> (2.75, 85.8349) projected
  line L525 (4, 85.5) -> (4, 84.7679) projected
  line L526 (2.75, 84.4329) -> (2.75, 83.8349) projected
  line L527 (4, 83.5) -> (4, 82.7679) projected
  line L528 (2.75, 82.4329) -> (2.75, 81.8349) projected
  line L529 (4, 81.5) -> (4, 80.7679) projected
  line L530 (2.75, 80.4329) -> (2.75, 79.8349) projected
  line L531 (4, 79.5) -> (4, 78.7679) projected
  line L532 (2.75, 78.4329) -> (2.75, 77.8349) projected
  line L533 (4, 77.5) -> (4, 76.7679) projected
  line L534 (2.75, 76.4329) -> (2.75, 75.8349) projected
  line L535 (4, 75.5) -> (4, 74.7679) projected
  line L536 (2.75, 74.4329) -> (2.75, 73.8349) projected
  line L537 (4, 73.5) -> (4, 72.7679) projected
  line L538 (2.75, 72.4329) -> (2.75, 71.8349) projected
  line L539 (4, 71.5) -> (4, 70.7679) projected
  line L540 (2.75, 70.4329) -> (2.75, 69.8349) projected
  line L541 (4, 69.5) -> (4, 68.7679) projected
  line L542 (2.75, 68.4329) -> (2.75, 67.8349) projected
  line L543 (4, 67.5) -> (4, 66.7679) projected
  line L544 (2.75, 66.4329) -> (2.75, 65.8349) projected
  line L545 (4, 65.5) -> (4, 64.7679) projected
  line L546 (2.75, 64.4329) -> (2.75, 63.8349) projected
  line L547 (4, 63.5) -> (4, 62.7679) projected
  line L548 (2.75, 62.4329) -> (2.75, 61.8349) projected
  line L549 (4, 61.5) -> (4, 60.7679) projected
  line L550 (2.75, 60.4329) -> (2.75, 59.8349) projected
  line L551 (4, 59.5) -> (4, 58.7679) projected
  line L552 (2.75, 58.4329) -> (2.75, 57.8349) projected
  line L553 (4, 57.5) -> (4, 56.7679) projected
  line L554 (2.75, 56.4329) -> (2.75, 55.8349) projected
  line L555 (4, 55.5) -> (4, 54.7679) projected
  line L556 (2.75, 54.4329) -> (2.75, 53.8349) projected
  line L557 (4, 53.5) -> (4, 52.7679) projected
  line L558 (2.75, 52.4329) -> (2.75, 51.8349) projected
  line L559 (4, 51.5) -> (4, 50.7679) projected
  line L560 (2.75, 50.4329) -> (2.75, 49.8349) projected
  line L561 (4, 49.5) -> (4, 48.7679) projected
  line L562 (2.75, 48.4329) -> (2.75, 47.8349) projected
  line L563 (4, 47.5) -> (4, 46.7679) projected
  line L564 (2.75, 46.4329) -> (2.75, 45.8349) projected
  line L565 (4, 45.5) -> (4, 44.7679) projected
  line L566 (2.75, 44.4329) -> (2.75, 43.8349) projected
  line L567 (4, 43.5) -> (4, 42.7679) projected
  line L568 (2.75, 42.4329) -> (2.75, 41.8349) projected
  line L569 (4, 41.5) -> (4, 40.7679) projected
  line L570 (2.75, 40.4329) -> (2.75, 39.8349) projected
  line L571 (4, 39.5) -> (4, 38.7679) projected
  line L572 (2.75, 38.4329) -> (2.75, 37.8349) projected
  line L573 (4, 37.5) -> (4, 36.7679) projected
  line L574 (2.75, 36.4329) -> (2.75, 35.8349) projected
  line L575 (4, 35.5) -> (4, 34.7679) projected
  line L576 (2.75, 34.4329) -> (2.75, 33.8349) projected
  line L577 (4, 33.5) -> (4, 32.7679) projected
  line L578 (2.75, 32.4329) -> (2.75, 31.8349) projected
  line L579 (4, 31.5) -> (4, 30.7679) projected
  line L580 (2.75, 30.4329) -> (2.75, 29.8349) projected
  line L581 (4, 29.5) -> (4, 28.7679) projected
  line L582 (2.75, 28.4329) -> (2.75, 27.8349) projected
  line L583 (4, 27.5) -> (4, 26.7679) projected
  line L584 (2.75, 26.4329) -> (2.75, 25.8349) projected
  line L585 (4, 25.5) -> (4, 24.7679) projected
  line L586 (2.75, 24.4329) -> (2.75, 23.8349) projected
  line L587 (4, 23.5) -> (4, 22.7679) projected
  line L588 (2.75, 22.4329) -> (2.75, 21.8349) projected
  line L589 (4, 21.5) -> (4, 20.7679) projected
  line L590 (2.75, 20.4329) -> (2.75, 19.8349) projected
  line L591 (4, 19.5) -> (4, 18.7679) projected
  line L592 (2.75, 18.4329) -> (2.75, 17.8349) projected
  line L593 (4, 17.5) -> (4, 16.7679) projected
  line L594 (2.75, 16.4329) -> (2.75, 15.8349) projected
  line L595 (4, 15.5) -> (4, 14.7679) projected
  line L596 (2.75, 14.4329) -> (2.75, 13.8349) projected
  line L597 (4, 13.5) -> (4, 12.7679) projected
  line L598 (2.75, 12.4329) -> (2.75, 11.8349) projected
  line L599 (4, 11.5) -> (4, 10.7679) projected
  line L600 (2.75, 10.4329) -> (2.75, 9.8349) projected
  line L601 (4, 9.5) -> (4, 8.7679) projected
  line L602 (2.75, 8.4329) -> (2.75, 7.8349) projected
  line L603 (4, 7.5) -> (4, 6.7679) projected
  line L604 (2.75, 6.4329) -> (2.75, 5.8349) projected
  line L605 (4, 5.5) -> (4, 4.7679) projected
  line L606 (2.75, 4.4329) -> (2.75, 3.8349) projected
  line L607 (4, 3.5) -> (4, 2.7679) projected
  line L608 (2.75, 2.4329) -> (2.75, 1.8349) projected
  line L609 (4, 1.5) -> (4, 0.7679) projected
  line L610 (-4, 0) -> (-4, 0.5) projected
  line L611 (-4, 1.7679) -> (-4, 2.5) projected
  line L612 (-4, 3.7679) -> (-4, 4.5) projected
  line L613 (-4, 5.7679) -> (-4, 6.5) projected
  line L614 (-4, 7.7679) -> (-4, 8.5) projected
  line L615 (-4, 9.7679) -> (-4, 10.5) projected
  line L616 (-4, 11.7679) -> (-4, 12.5) projected
  line L617 (-4, 13.7679) -> (-4, 14.5) projected
  line L618 (-4, 15.7679) -> (-4, 16.5) projected
  line L619 (-4, 17.7679) -> (-4, 18.5) projected
  line L620 (-4, 19.7679) -> (-4, 20.5) projected
  line L621 (-4, 21.7679) -> (-4, 22.5) projected
  line L622 (-4, 23.7679) -> (-4, 24.5) projected
  line L623 (-4, 25.7679) -> (-4, 26.5) projected
  line L624 (-4, 27.7679) -> (-4, 28.5) projected
  line L625 (-4, 29.7679) -> (-4, 30.5) projected
  line L626 (-4, 31.7679) -> (-4, 32.5) projected
  line L627 (-4, 33.7679) -> (-4, 34.5) projected
  line L628 (-4, 35.7679) -> (-4, 36.5) projected
  line L629 (-4, 37.7679) -> (-4, 38.5) projected
  line L630 (-4, 39.7679) -> (-4, 40.5) projected
  line L631 (-4, 41.7679) -> (-4, 42.5) projected
  line L632 (-4, 43.7679) -> (-4, 44.5) projected
  line L633 (-4, 45.7679) -> (-4, 46.5) projected
  line L634 (-4, 47.7679) -> (-4, 48.5) projected
  line L635 (-4, 49.7679) -> (-4, 50.5) projected
  line L636 (-4, 51.7679) -> (-4, 52.5) projected
  line L637 (-4, 53.7679) -> (-4, 54.5) projected
  line L638 (-4, 55.7679) -> (-4, 56.5) projected
  line L639 (-4, 57.7679) -> (-4, 58.5) projected
  line L640 (-4, 59.7679) -> (-4, 60.5) projected
  line L641 (-4, 61.7679) -> (-4, 62.5) projected
  line L642 (-4, 63.7679) -> (-4, 64.5) projected
  line L643 (-4, 65.7679) -> (-4, 66.5) projected
  line L644 (-4, 67.7679) -> (-4, 68.5) projected
  line L645 (-4, 69.7679) -> (-4, 70.5) projected
  line L646 (-4, 71.7679) -> (-4, 72.5) projected
  line L647 (-4, 73.7679) -> (-4, 74.5) projected
  line L648 (-4, 75.7679) -> (-4, 76.5) projected
  line L649 (-4, 77.7679) -> (-4, 78.5) projected
  line L650 (-4, 79.7679) -> (-4, 80.5) projected
  line L651 (-4, 81.7679) -> (-4, 82.5) projected
  line L652 (-4, 83.7679) -> (-4, 84.5) projected
  line L653 (-4, 85.7679) -> (-4, 86.5) projected
  line L654 (-4, 87.7679) -> (-4, 88.5) projected
  line L655 (-4, 89.7679) -> (-4, 90.5) projected
  line L656 (-4, 91.7679) -> (-4, 92.5) projected
  line L657 (-4, 93.7679) -> (-4, 94.5) projected
  line L658 (-4, 95.7679) -> (-4, 96.5) projected
  line L659 (-4, 97.7679) -> (-4, 98.5) projected
  line L660 (-4, 99.7679) -> (-4, 100.5) projected
  line L661 (-4, 101.7679) -> (-4, 102.5) projected
  line L662 (-4, 103.7679) -> (-4, 104.5) projected
  line L663 (-4, 105.7679) -> (-4, 106.5) projected
  line L664 (-4, 107.7679) -> (-4, 108.5) projected
  line L665 (-4, 109.7679) -> (-4, 110.5) projected
  line L666 (-4, 111.7679) -> (-4, 112.5) projected
  line L667 (-4, 113.7679) -> (-4, 114.5) projected
  line L668 (-4, 115.7679) -> (-4, 116.5) projected
  line L669 (-4, 117.7679) -> (-4, 118.5) projected
  line L670 (-4, 119.7679) -> (-4, 120.5) projected
  line L671 (-4, 121.7679) -> (-4, 122.5) projected
  line L672 (-4, 123.7679) -> (-4, 124.5) projected
  line L673 (-4, 125.7679) -> (-4, 126.5) projected
  line L674 (-4, 127.7679) -> (-4, 128.5) projected
  line L675 (-4, 129.7679) -> (-4, 130.5) projected
  line L676 (-4, 131.7679) -> (-4, 132.5) projected
  line L677 (-4, 133.7679) -> (-4, 134.5) projected
  line L678 (-4, 135.7679) -> (-4, 136.5) projected
  line L679 (-4, 137.7679) -> (-4, 138.5) projected
  line L680 (-4, 139.7679) -> (-4, 140.5) projected
  line L681 (-4, 141.7679) -> (-4, 142.5) projected
  line L682 (-4, 143.7679) -> (-4, 144.5) projected
  line L683 (-4, 145.7679) -> (-4, 146.5) projected
  line L684 (-4, 147.7679) -> (-4, 148.5) projected
  line L685 (-4, 149.7679) -> (-4, 150.5) projected
  line L686 (-4, 151.7679) -> (-4, 152.5) projected
  line L687 (-4, 153.7679) -> (-4, 154.5) projected
  line L688 (-4, 155.7679) -> (-4, 156.5) projected
  line L689 (-4, 157.7679) -> (-4, 158.5) projected
  line L690 (-4, 159.7679) -> (-4, 160.5) projected
  line L691 (-4, 161.7679) -> (-4, 162.5) projected
  line L692 (-4, 163.7679) -> (-4, 164.5) projected
  line L693 (-4, 165.7679) -> (-4, 166.5) projected
  line L694 (-4, 167.7679) -> (-4, 168.5) projected
  line L695 (-4, 169.7679) -> (-4, 170.5) projected
  line L696 (-4, 171.7679) -> (-4, 172.5) projected
  line L697 (-4, 173.7679) -> (-4, 174.5) projected
  line L698 (-4, 175.7679) -> (-4, 176.5) projected
  line L699 (-4, 177.7679) -> (-4, 178.5) projected
  line L700 (-4, 179.7679) -> (-4, 180.5) projected
  line L701 (-4, 181.7679) -> (-4, 182.5) projected
  line L702 (-4, 183.7679) -> (-4, 184.5) projected
  line L703 (-4, 185.7679) -> (-4, 186.5) projected
  line L704 (-4, 187.7679) -> (-4, 188.5) projected
  line L705 (-4, 189.7679) -> (-4, 190.5) projected
  line L706 (-4, 191.7679) -> (-4, 192.5) projected
  line L707 (-4, 193.7679) -> (-4, 194.5) projected
  line L708 (-4, 195.7679) -> (-4, 196.5) projected
  line L709 (-4, 197.7679) -> (-4, 198.5) projected
  line L710 (-4, 199.7679) -> (-4, 200.5) projected
  line L711 (-4, 201.7679) -> (-4, 202.5) projected
  line L712 (-4, 203.7679) -> (-4, 204.5) projected
  line L713 (-4, 205.7679) -> (-4, 206.5) projected
  line L714 (-4, 207.7679) -> (-4, 208.5) projected
  line L715 (-4, 209.7679) -> (-4, 210.5) projected
  line L716 (-4, 211.7679) -> (-4, 212.5) projected
  line L717 (-4, 213.7679) -> (-4, 214.5) projected
  line L718 (-4, 215.7679) -> (-4, 216.5) projected
  line L719 (-4, 217.7679) -> (-4, 218.5) projected
  line L720 (-4, 219.7679) -> (-4, 220.5) projected
  line L721 (-4, 221.7679) -> (-4, 222.5) projected
  line L722 (-4, 223.7679) -> (-4, 224.5) projected
  line L723 (-4, 225.7679) -> (-4, 226.5) projected
  line L724 (-4, 227.7679) -> (-4, 228.5) projected
  line L725 (-4, 229.7679) -> (-4, 230.5) projected
  line L726 (-4, 231.7679) -> (-4, 232.5) projected
  line L727 (-4, 233.7679) -> (-4, 234.5) projected
  line L728 (-4, 235.7679) -> (-4, 236.5) projected
  line L729 (-4, 237.7679) -> (-4, 238.5) projected
  line L730 (-4, 239.7679) -> (-4, 240.5) projected
  line L731 (-4, 241.7679) -> (-4, 242.5) projected
  line L732 (-4, 243.7679) -> (-4, 244.5) projected
  line L733 (-4, 245.7679) -> (-4, 246.5) projected
  line L734 (-4, 247.7679) -> (-4, 248.5) projected
  line L735 (-4, 249.7679) -> (-4, 250.5) projected
  line L736 (-4, 251.7679) -> (-4, 252.5) projected
  line L737 (-4, 253.7679) -> (-4, 254.5) projected
  line L738 (-4, 255.7679) -> (-4, 256.5) projected
  line L739 (-4, 257.7679) -> (-4, 258.5) projected
  line L740 (-4, 259.7679) -> (-4, 260.5) projected
  line L741 (-4, 261.7679) -> (-4, 262.5) projected
  line L742 (-4, 263.7679) -> (-4, 264.5) projected
  line L743 (-4, 265.7679) -> (-4, 266.5) projected
  line L744 (-4, 267.7679) -> (-4, 268.5) projected
  line L745 (-4, 269.7679) -> (-4, 270.5) projected
  line L746 (-4, 271.7679) -> (-4, 272.5) projected
  line L747 (-4, 273.7679) -> (-4, 274.5) projected
  line L748 (-4, 275.7679) -> (-4, 276.5) projected
  line L749 (-4, 277.7679) -> (-4, 278.5) projected
  line L750 (-4, 279.7679) -> (-4, 280.5) projected
  line L751 (-4, 281.7679) -> (-4, 282.5) projected
  line L752 (-4, 283.7679) -> (-4, 284.5) projected
  line L753 (-4, 285.7679) -> (-4, 286.5) projected
  line L754 (-4, 287.7679) -> (-4, 288.5) projected
  line L755 (-4, 289.7679) -> (-4, 290.5) projected
  line L756 (-4, 291.7679) -> (-4, 292.5) projected
  line L757 (-4, 293.7679) -> (-4, 294.5) projected
  line L758 (-4, 295.7679) -> (-4, 296.5) projected
  line L759 (-4, 297.7679) -> (-4, 298.5) projected
  line L760 (-4, 299.7679) -> (-4, 300.5) projected
  line L761 (-4, 301.7679) -> (-4, 302.5) projected
  line L762 (-4, 303.7679) -> (-4, 304.5) projected
  line L763 (-4, 305.7679) -> (-4, 306.5) projected
  line L764 (-4, 307.7679) -> (-4, 308.5) projected
  line L765 (-4, 309.7679) -> (-4, 310.5) projected
  line L766 (-4, 311.7679) -> (-4, 312.5) projected
  line L767 (-4, 313.7679) -> (-4, 314.5) projected
  line L768 (-4, 315.7679) -> (-4, 316.5) projected
  line L769 (-4, 317.7679) -> (-4, 318.5) projected
  line L770 (-4, 319.7679) -> (-4, 320.5) projected
  line L771 (-4, 321.7679) -> (-4, 322.5) projected
  line L772 (-4, 323.7679) -> (-4, 324.5) projected
  line L773 (-4, 325.7679) -> (-4, 326.5) projected
  line L774 (-4, 327.7679) -> (-4, 328.5) projected
  line L775 (-4, 329.7679) -> (-4, 330.5) projected
  line L776 (-4, 331.7679) -> (-4, 332.5) projected
  line L777 (-4, 333.7679) -> (-4, 334.5) projected
  line L778 (-4, 335.7679) -> (-4, 336.5) projected
  line L779 (-4, 337.7679) -> (-4, 338.5) projected
  line L780 (-4, 339.7679) -> (-4, 340.5) projected
  line L781 (-4, 341.7679) -> (-4, 342.5) projected
  line L782 (-4, 343.7679) -> (-4, 344.5) projected
  line L783 (-4, 345.7679) -> (-4, 346.5) projected
  line L784 (-4, 347.7679) -> (-4, 348.5) projected
  line L785 (-4, 349.7679) -> (-4, 350.5) projected
  line L786 (-4, 351.7679) -> (-4, 352.5) projected
  line L787 (-4, 353.7679) -> (-4, 354.5) projected
  line L788 (-4, 355.7679) -> (-4, 356.5) projected
  line L789 (-4, 357.7679) -> (-4, 358.5) projected
  line L790 (-4, 359.7679) -> (-4, 360.5) projected
  line L791 (-4, 361.7679) -> (-4, 362.5) projected
  line L792 (-4, 363.7679) -> (-4, 364.5) projected
  line L793 (-4, 365.7679) -> (-4, 366.5) projected
  line L794 (-4, 367.7679) -> (-4, 368.5) projected
  line L795 (-4, 369.7679) -> (-4, 370.5) projected
  line L796 (-4, 371.7679) -> (-4, 372.5) projected
  line L797 (-4, 373.7679) -> (-4, 374.5) projected
  line L798 (-4, 375.7679) -> (-4, 376.5) projected
  line L799 (-4, 377.7679) -> (-4, 378.5) projected
  line L800 (-4, 379.7679) -> (-4, 380.5) projected
  line L801 (-4, 381.7679) -> (-4, 382.5) projected
  line L802 (-4, 383.7679) -> (-4, 384.5) projected
  line L803 (-4, 385.7679) -> (-4, 386.5) projected
  line L804 (-4, 387.7679) -> (-4, 388.5) projected
  line L805 (-4, 389.7679) -> (-4, 390.5) projected
  line L806 (-4, 391.7679) -> (-4, 392.5) projected
  line L807 (-4, 393.7679) -> (-4, 394.5) projected
  line L808 (-4, 395.7679) -> (-4, 396.5) projected
  line L809 (-4, 397.7679) -> (-4, 398.5) projected
  line L810 (-4.0034, 400.9402) -> (-4.0034, 400.3422)
  line L811 (-4.0034, 400.9402) -> (-2.7534, 401.2752)
  line L812 (-2.7534, 401.2752) -> (-2.7534, 400.0073)
  line L813 (-2.7534, 400.6412) -> (-4.0034, 400.6412) construction
  line L814 (-4.0034, 400.3422) -> (-2.7534, 400.0073)
  point P0 (0, 0)
  dimension "d30" = 1.25
  constraints: 22 end point, 6 symmetric about line, 2 midpoint, 1 vertical, 800 other
  measures "d30" distance of L204.start L204.end
equation "\"d8\" = 0.634 * pitch - 0.536 * di"
equation "\"d13\" = pitch"
equation "\"d30\" = di"
equation "\"pitch\" = 2"
body "Solid1"
